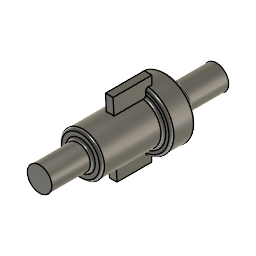
Cotter Joint (2) (Autodesk Fusion 360 design; units mm, degrees)
Autodesk Fusion 360 part; units mm, degrees
sketch "Sketch1" plane through (0, 0, 0) normal (0, 1, 0) x (1, 0, 0)
  circle A0 centre (0, 0) radius 15
  circle A1 centre (0, 0) radius 22.5
  dimension "d1" = 30
  dimension "d4" = 45
  constraint coincident A0.centre A1.centre
  constraint concentric A0 A1
  measures "d1" diameter of A0
  measures "d4" diameter of A1
extrude "Extrude1" add sketch "Sketch1" along normal blind 50 contours A0 makes body 1
extrude "Extrude2" add sketch "Sketch1" against normal blind 11 separate body contours A0 | A1 makes body 2
sketch "Sketch2" plane through (0, -11, 0) normal (0, -1, 0) x (1, 0, 0)
  circle A0 centre (0, 0) radius 22.5
  circle A1 centre (0, 0) radius 18
  dimension "d7" = 36
  constraint coincident A0.centre A1.centre
  measures "d7" diameter of A1
extrude "Extrude3" add sketch "Sketch2" along normal blind 90 contours A1 bodies 2
combine "Combine1" operation add target body 1 tool bodies 2
copy_body "Body->Comp1" bodies 1 removing the originals makes body 3 in component "spigot"
sketch "Sketch3" plane through (0, 0, 0) normal (0, 1, 0) x (1, 0, 0)
  circle A0 centre (0, 0) radius 15
  circle A1 centre (0, 0) radius 26.25
  dimension "d11" = 30
  dimension "d14" = 52.5
  constraint coincident A0.centre A1.centre
  constraint concentric A0 A1
  measures "d11" diameter of A0
  measures "d14" diameter of A1
extrude "Extrude4" add sketch "Sketch3" against normal blind 50 separate body contours A0 makes body 4
extrude "Extrude5" add sketch "Sketch3" along normal blind 105 contours A0 | A1 bodies 4
sketch "Sketch4" plane through (0, 105, 0) normal (0, 1, 0) x (-1, 0, 0)
  circle A0 centre (0, 0) radius 26.25
  circle A1 centre (0, 0) radius 36
  dimension "d17" = 72
  constraint coincident A0.centre A1.centre
  measures "d17" diameter of A1
extrude "Extrude6" add sketch "Sketch4" against normal blind 30 bodies 4
sketch "Sketch5" plane through (0, 105, 0) normal (0, 1, 0) x (-1, 0, 0)
  circle A0 centre (0, 0) radius 36
  circle A1 centre (0, 0) radius 18
  dimension "d20" = 36
  constraint coincident A0.centre A1.centre
  measures "d20" diameter of A1
extrude "Extrude7" cut sketch "Sketch5" against normal blind 90 contours A1 bodies 4
fillet "Fillet1" radius 3 1 edges at (16.7819, 15, 6.5091) on bodies 4
fillet "Fillet1'" radius 3 1 edges at (-16.7819, -101, -6.5091) on bodies 3 in component "spigot"
fillet "Fillet2" radius 3 1 edges at (-24.4736, 0, 9.4924) on bodies 4
fillet "Fillet2'" radius 3 1 edges at (-20.9774, 0, 8.1363) on bodies 3 in component "spigot"
fillet "Fillet2'" radius 3 1 edges at (-20.9774, -11, -8.1363) on bodies 3 in component "spigot"
fillet "Fillet3" radius 3 3 edges at (33.5638, 105, -13.0182) (33.5638, 75, 13.0182) (-13.9849, 0, 5.4242) on bodies 4
fillet "Fillet3" radius 3 1 edges at (-24.4736, 75, -9.4924) on bodies 4
sketch "Sketch6" plane through (0, 0, 0) normal (1, 0, 0) x (0, 1, 0)
  line L0 (75, -33) -> (75, -29.25)
  line L1 (75, 29.25) -> (75, 33)
  line L2 (0, 18) -> (0, 23.25)
  line L3 (0, -23.25) -> (0, -18)
  line L4 (-50, 0) -> (-50, -15)
  line L5 (-50, 15) -> (-50, 0)
  line L6 (105, 33) -> (105, -33)
  arc A0 (75, -29.25) -> (72, -26.25) centre (72, -29.25) ccw
  arc A1 (72, 26.25) -> (75, 29.25) centre (72, 29.25) ccw
  line L7 (3, -26.25) -> (72, -26.25)
  line L8 (3, 26.25) -> (72, 26.25)
  arc A2 (-3, 15) -> (0, 18) centre (-3, 18) ccw
  arc A3 (0, -18) -> (-3, -15) centre (-3, -18) ccw
  line L9 (-3, 15) -> (-50, 15)
  line L10 (-3, -15) -> (-50, -15)
  arc A4 (75, -33) -> (78, -36) centre (78, -33) ccw
  arc A5 (78, 36) -> (75, 33) centre (78, 33) ccw
  line L11 (102, 36) -> (78, 36)
  line L12 (102, -36) -> (78, -36)
  arc A6 (105, 33) -> (102, 36) centre (102, 33) ccw
  arc A7 (102, -36) -> (105, -33) centre (102, -33) ccw
  arc A8 (3, 26.25) -> (0, 23.25) centre (3, 23.25) ccw
  arc A9 (0, -23.25) -> (3, -26.25) centre (3, -23.25) ccw
  line L13 (-50, 0) -> (109.5, 0) construction
  line L14 (82.5, 46) -> (82.5, -46)
  line L15 (82.5, 0) -> (37.5, 0)
  line L16 (37.5, 0) -> (35.0892, 46)
  line L17 (82.5, 46) -> (35.0892, 46)
  line L18 (82.5, -46) -> (39.9108, -46)
  line L19 (37.5, 0) -> (39.9108, -46)
  point P0 (82.5, -46)
  point P1 (82.5, 46)
  dimension "d41" = 22.5
  dimension "d42" = 45
  dimension "d43" = 93
  dimension "d44" = 92
  constraint coincident L4.start L5.end
  constraint perpendicular L4 L13
  constraint perpendicular L12 L14
  constraint symmetric L13 P1 P0
  constraint symmetric L13 P0 P1
  constraint coincident L13 L15.start
  constraint coincident L14 L15.start
  constraint coincident L13 L15.end
  constraint perpendicular L14 L17
  constraint coincident P0 L14.end
  constraint horizontal L18
  constraint parallel L16 L19
  measures "d41" distance of L6 L14
  measures "d42" distance of L15.start L15.end
  measures "d43" angle of L13 L16
  measures "d44" distance of P1 P0
extrude "Extrude8" add sketch "Sketch6" along normal mid plane 9.3 separate body contours L0 A0 L7 A4 L12 L14 L18 L19 | L0 A0 L7 A4 L12 L14 L15 L19 | L1 A1 L8 A5 L11 L14 L15 L16 | L1 A1 L8 A5 L11 L14 L16 L17 makes body 5
combine "Combine2" operation cut target body 4 tool bodies 5 keep tools
combine "Combine1'" operation cut target body 3 tool bodies 5 body 5 seen with x (1, 0, 0) y (0, 1, 0) z (0, 0, 1) at (0, -116, 0) keep tools in component "spigot"
component "spigot" placed x (1, 0, 0) y (0, 1, 0) z (0, 0, 1) at (0, 116, 0)
named bodies: "spigot", "Socket", "Cotter"
